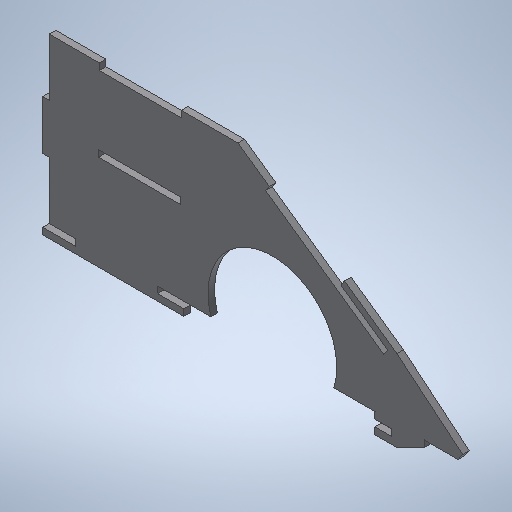
# Autodesk Inventor part: Tapa lateral 1
Saved by Autodesk Inventor 2025 (Build 290162000, 162)
## iProperties
Created: 2024-10-18
Part Number: Tapa lateral 1
Material: Generic
Document SubType Name: Modeling
Designer: feder
Density: 1 g/cm^3
Appearance: Default
Author: feder
Autodesk Inventor part; units mm, degrees
ref_plane "YZ Plane" through (0, 0, 0) normal (1, 0, 0) x (0, 1, 0)
ref_plane "XZ Plane" through (0, 0, 0) normal (0, 1, 0) x (-1, 0, 0)
ref_plane "XY Plane" through (0, 0, 0) normal (0, 0, 1) x (1, 0, 0)
sketch "Sketch1" plane through (0, 0, 0) normal (0, 0, 1) x (1, 0, 0)
  line L0 (-100, 100) -> (100, 100)
  line L1 (100, 100) -> (100, 0)
  line L2 (100, 0) -> (-100, 0)
  line L3 (-100, 0) -> (-100, 100)
  arc A0 (77.5, 0) -> (2.5, 0) centre (40, 11.6402) ccw
  point P0 (0, 0)
  point P1 (0, 100)
  point P2 (0, 0)
  dimension "d0" = 200
  dimension "d1" = 100
  dimension "d22" = 75
  dimension "d23" = 102.5
  constraints: 8 end point, 2 midpoint, 2 parallel, 2 point on circle, 2 point on line, 1 centre point, 1 coincident, 1 horizontal, 1 perpendicular, 1 vertical alignment
  measures "d0" distance of L0.start L0.end
  measures "d1" distance of L0.end L1.end
  measures "d22" distance of A0.end A0.start
  measures "d23" distance from line of L3 A0.end
extrude "Extrusion1" add sketch "Sketch1" along normal blind 4 contours L0 L1 L2 A0 L3
sketch "Sketch2" plane through (0, 0, 4) normal (0, 0, 1) x (1, 0, 0)
  line L0 (-100, 100) -> (-100, 0) projected
  line L1 (-100, 0) -> (-96, 0)
  line L2 (-96, 0) -> (-96, 35)
  line L3 (-96, 35) -> (-100, 35)
  line L4 (-100, 35) -> (-100, 0)
  line L5 (-100, 100) -> (-96, 100)
  line L6 (-96, 100) -> (-96, 65)
  line L7 (-96, 65) -> (-100, 65)
  line L8 (-100, 65) -> (-100, 100)
  point P0 (0, 0)
  dimension "d9" = 4
  dimension "d10" = 35
  dimension "d11" = 4
  dimension "d12" = 35
  constraints: 16 end point, 4 parallel, 2 horizontal, 2 perpendicular
  measures "d9" distance of L2.end L3.end
  measures "d10" distance of L1.end L2.end
  measures "d11" distance of L6.end L7.end
  measures "d12" distance of L5.end L6.end
extrude "Extrusion2" cut sketch "Sketch2" against normal through all
sketch "Sketch3" plane through (-24.1746, 0, 0) normal (0, -1, 0) x (1, 0, 0)
  line L0 (-71.8254, 4) -> (124.1746, 4) projected
  line L1 (-55.8254, 4) -> (-5.8254, 4)
  line L2 (-5.8254, 4) -> (-5.8254, 0)
  line L3 (-5.8254, 0) -> (-55.8254, 0)
  line L4 (-55.8254, 0) -> (-55.8254, 4)
  line L5 (-75.8254, 0) -> (-75.8254, 4) projected
  line L6 (124.1746, 0) -> (-71.8254, 0) projected
  line L7 (124.1746, 4) -> (-71.8254, 4) projected
  line L8 (124.1746, 0) -> (124.1746, 4) projected
  point P0 (24.1746, 0)
  point P1 (0, 4)
  point P2 (117.1746, 0)
  point P3 (105.1746, 4)
  point P4 (-5.8254, 4)
  dimension "d15" = 4
  dimension "d16" = 20
  dimension "d17" = 50
  constraints: 8 end point, 3 point on line, 2 parallel, 1 horizontal, 1 perpendicular
  measures "d15" distance of L3.end L1.start
  measures "d16" distance between parallel lines of L5 L4
  measures "d17" distance between parallel lines of L2 L4
extrude "Extrusion3" add sketch "Sketch3" along normal blind 4 contours L0 L2 L3 L4
sketch "Sketch5" plane through (100, 0, 0) normal (1, 0, 0) x (0, 0, -1)
  line L0 (-4, 100) -> (-4, 65) projected
  line L1 (-4, 100) -> (0, 100)
  line L2 (0, 100) -> (0, 0)
  line L3 (0, 0) -> (-4, 0)
  line L4 (-4, 0) -> (-4, 100)
  constraints: 8 end point, 2 parallel, 1 horizontal, 1 perpendicular
extrude "Extrusion5" add sketch "Sketch5" along normal blind 80
sketch "Sketch6" plane through (0, 0, 4) normal (0, 0, 1) x (1, 0, 0)
  line L0 (-96, 100) -> (180, 100) projected
  line L1 (180, 100) -> (19, 100)
  line L2 (180, 100) -> (180, 0) projected
  line L3 (180, 100) -> (180, -12.7334)
  line L4 (180, -12.7334) -> (19, 100)
  point P0 (0, 0)
  dimension "d30" = 35
  dimension "d33" = 115
  constraints: 6 end point, 2 point on line
  measures "d30" angle of L4 L0
  measures "d33" distance of L0.start L1.end
extrude "Extrusion6" cut sketch "Sketch6" against normal blind 80
sketch "Sketch7" plane through (161.8148, 0, 4) normal (0.5735764, 0.819152, 0) x (0.819152, -0.5735764, 0)
  line L0 (0, 0) -> (-174.3447, 0) projected
  line L1 (-69.0666, 4) -> (-145.7265, 4) projected
  line L2 (-63, 0) -> (-113, 0)
  line L3 (-113, 0) -> (-113, 4)
  line L4 (-113, 4) -> (-63, 4)
  line L5 (-63, 4) -> (-63, 0)
  line L6 (0, 4) -> (0, 0) projected
  line L7 (-113, 0) -> (-151, 0)
  line L8 (-151, 0) -> (-151, 4)
  line L9 (-151, 4) -> (-113, 4)
  line L10 (-113, 4) -> (-113, 0)
  point P0 (-132.5509, 4)
  point P1 (-130.503, 4)
  point P2 (0, 2)
  point P3 (-63, 2)
  point P4 (-113, 0)
  point P5 (-151, 0)
  dimension "d34" = 50
  dimension "d35" = 63
  dimension "d56" = 38
  constraints: 16 end point, 4 parallel, 3 point on line, 2 horizontal, 2 midpoint, 2 perpendicular
  measures "d34" distance between parallel lines of L5 L3
  measures "d35" distance of point (0, 2) point (-63, 2)
  measures "d56" distance between parallel lines of L3 L8
extrude "Extrusion7" cut sketch "Sketch7" against normal blind 4
sketch "Sketch8" plane through (-96, 100, 4) normal (0, 1, 0) x (1, 0, 0)
  line L0 (112, 4) -> (0, 4)
  line L1 (63, 0) -> (80.5, 0)
  line L2 (30.5, 4) -> (80.5, 4)
  line L3 (80.5, 4) -> (80.5, 0)
  line L4 (80.5, 0) -> (30.5, 0)
  line L5 (30.5, 0) -> (30.5, 4)
  line L6 (0, 4) -> (0, 0)
  line L7 (0, 4) -> (0, 0) projected
  point P0 (96, 4)
  point P1 (80.5, 2)
  point P2 (30.5, 2)
  point P3 (80.5, 4)
  point P4 (0, 2)
  point P5 (0, 2)
  dimension "d38" = 50
  dimension "d42" = 30.5
  constraints: 14 end point, 4 midpoint, 1 point on line
  measures "d38" distance of point (80.5, 2) point (30.5, 2)
  measures "d42" distance of point (30.5, 2) point (0, 2)
extrude "Extrusion8" cut sketch "Sketch8" against normal blind 4
sketch "Sketch9" plane through (161.8148, 0, 4) normal (0.5735764, 0.819152, 0) x (0.819152, -0.5735764, 0)
  line L0 (-63, 4) -> (0, 4) projected
  line L1 (0, 0) -> (-63, 0) projected
  line L2 (0, 4) -> (-7.082, 4)
  line L3 (-7.082, 4) -> (-7.082, 0)
  line L4 (-7.082, 0) -> (0, 0)
  line L5 (0, 0) -> (0, 4)
  point P0 (-132.5509, 4)
  point P1 (-7.082, 4)
  dimension "d43" = 7.082
  constraints: 8 end point, 2 parallel, 1 horizontal, 1 perpendicular, 1 point on line
  measures "d43" distance of L4.end L3.end
extrude "Extrusion9" cut sketch "Sketch9" against normal through all
sketch "Sketch10" plane through (77.5, 0, 0) normal (0, -1, 0) x (1, 0, 0)
  line L0 (30.4139, 4) -> (-41.6715, 4) projected
  line L1 (32.7082, 0) -> (78.5136, 0) projected
  line L2 (25, 4) -> (55, 4)
  line L3 (55, 4) -> (55, 0)
  line L4 (55, 0) -> (25, 0)
  line L5 (25, 0) -> (25, 4)
  line L6 (0, 0) -> (0, 4) projected
  point P0 (-77.5, 0)
  point P1 (-10.5437, 4)
  point P2 (25, 2)
  point P3 (0, 2)
  dimension "d46" = 30
  dimension "d47" = 25
  constraints: 8 end point, 2 midpoint, 2 parallel, 2 point on line, 1 horizontal, 1 perpendicular
  measures "d46" distance between parallel lines of L3 L5
  measures "d47" distance of point (25, 2) point (0, 2)
extrude "Extrusion10" add sketch "Sketch10" along normal blind 4
sketch "Sketch11" plane through (0, 0, 0) normal (0, 0, -1) x (-1, 0, 0)
  line L0 (16, 54) -> (66, 54)
  line L1 (66, 54) -> (66, 50)
  line L2 (66, 50) -> (16, 50)
  line L3 (16, 50) -> (16, 54)
  line L4 (96, 0) -> (96, 35) projected
  point P0 (0, 0)
  point P1 (41, 50)
  dimension "d50" = 50
  dimension "d51" = 4
  dimension "d52" = 55
  dimension "d53" = 50
  constraints: 8 end point, 2 parallel, 1 horizontal, 1 midpoint, 1 perpendicular
  measures "d50" distance of L0.start L0.end
  measures "d51" distance of L0.end L1.end
  measures "d52" distance from line of L4 point (41, 50)
  measures "d53" distance from line of L2 point (0, 0)
extrude "Extrusion11" cut sketch "Sketch11" against normal blind 4
sketch "Sketch15" plane through (0, 0, 4) normal (0, 0, 1) x (1, 0, 0)
  line L0 (107.9139, 32.8587) -> (35.8285, 83.3334) projected
  line L1 (107.9139, 32.8587) -> (100.9511, 37.7341)
  line L2 (110.2082, 36.1353) -> (107.9139, 32.8587) projected
  line L3 (107.9139, 32.8587) -> (112.6172, 39.5758)
  line L4 (110.2082, 36.1353) -> (113.4848, 33.841)
  line L5 (156.0136, 4.0621) -> (110.2082, 36.1353) projected
  line L6 (112.6172, 39.5758) -> (115.8939, 37.2814)
  line L7 (115.8939, 37.2814) -> (113.4848, 33.841)
  line L8 (112.6172, 39.5758) -> (83.9469, 59.6509)
  line L9 (83.9469, 59.6509) -> (81.6526, 56.3743)
  line L10 (81.6526, 56.3743) -> (110.3229, 36.2991)
  line L11 (115.8939, 37.2814) -> (156.0136, 4.0621)
  point P0 (0, 0)
  point P1 (120.2672, 29.092)
  dimension "d61" = 8.2
  dimension "d62" = 4
  dimension "d63" = 35
  dimension "d64" = 4
  constraints: 18 end point, 8 point on line, 3 perpendicular, 1 collinear
  measures "d61" distance of L3.start L3.end
  measures "d62" distance of L2.start L4.end
  measures "d63" distance of L3.end L8.end
  measures "d64" distance of L8.end L9.end
extrude "Extrusion12" add sketch "Sketch15" against normal blind 4
sketch "Sketch16" plane through (77.5, -4, 0) normal (0, -1, 0) x (1, 0, 0)
  line L0 (55, 0) -> (55, 4) projected
  line L1 (25, 0) -> (55, 0) projected
  line L2 (55, 4) -> (25, 4)
  line L3 (25, 4) -> (25, 0)
  line L4 (25, 0) -> (55, 0)
  line L5 (55, 0) -> (55, 4)
  point P0 (-77.5, 0)
  constraints: 8 end point, 2 parallel, 1 horizontal, 1 perpendicular
extrude "Extrusion13" add sketch "Sketch16" along normal blind 8.3
sketch "Sketch17" plane through (0, 0, 4) normal (0, 0, 1) x (1, 0, 0)
  line L0 (77.5, 0) -> (102.5, 0) projected
  line L1 (102.5, 0) -> (102.5, -12.3) projected
  line L2 (102.5, -4) -> (112.5, -4)
  line L3 (112.5, -4) -> (112.5, -8.1)
  line L4 (112.5, -8.1) -> (102.5, -8.1)
  line L5 (102.5, -8.1) -> (102.5, -4)
  line L6 (132.5, -12.3) -> (102.5, -12.3) projected
  line L7 (117.5, -12.3) -> (132.5, -12.3)
  line L8 (132.5, -12.3) -> (132.5, 0)
  line L9 (132.5, -4) -> (116.0511, -12.3)
  point P0 (0, 0)
  dimension "d71" = 4
  dimension "d72" = 4.1
  dimension "d73" = 4.2
  dimension "d74" = 10
  dimension "d77" = 4
  constraints: 14 end point, 3 point on line, 2 horizontal, 2 parallel, 2 perpendicular, 1 midpoint
  measures "d71" distance from line of L2 L0.end
  measures "d72" distance between parallel lines of L4 L2
  measures "d73" distance between parallel lines of L6 L4
  measures "d74" distance between parallel lines of L1 L3
  measures "d77" distance of L8.end L9.start
extrude "Extrusion14" cut sketch "Sketch17" against normal blind 8.3
sketch "Sketch21" plane through (0, 0, 4) normal (0, 0, 1) x (1, 0, 0)
  line L0 (-80, -4) -> (-100, -4)
  line L1 (-100, -4) -> (-100, -8)
  line L2 (-100, -8) -> (-80, -8)
  line L3 (-80, -8) -> (-80, -4)
  line L4 (-80, -4) -> (-30, -4)
  line L5 (-30, -4) -> (-30, -8)
  line L6 (-30, -8) -> (-80, -8)
  line L7 (-80, -8) -> (-80, -4)
  line L8 (-30, -4) -> (-30, -4)
  line L9 (-30, -8) -> (-14, -8)
  line L10 (-30, -4) -> (-14, -4)
  line L11 (-14, -4) -> (-14, -8)
  line L12 (-14, -8) -> (-30, -8)
  line L13 (-30, -8) -> (-30, -4)
  point P0 (0, 0)
  dimension "d80" = 20
  dimension "d81" = 4
  dimension "d82" = 50
  dimension "d85" = 16
  constraints: 28 end point, 6 parallel, 4 horizontal, 3 perpendicular, 1 collinear
  measures "d80" distance of L2.end L1.end
  measures "d81" distance of L0.end L1.end
  measures "d82" distance of L5.end L6.end
  measures "d85" distance of L5.end L9.end
extrude "Extrusion15" add sketch "Sketch21" against normal blind 4
body "Solid1"
